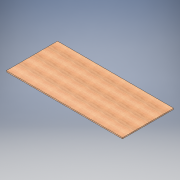
# Autodesk Inventor part: BedSlat
Saved by Autodesk Inventor 2017 (Build 210142000, 142)
## iProperties
Created: 2016-10-24
Part Number: BedSlat
Material: Generic
Document SubType Name: Modeling
Designer: andrew
Density: 1 g/cm^3
Appearance: Birch - Natural Polished
d1: 80.000 in
d2: 35.250 in
Author: andrew
Autodesk Inventor part; units mm, degrees
ref_plane "YZ Plane" through (0, 0, 0) normal (1, 0, 0) x (0, 1, 0)
ref_plane "XZ Plane" through (0, 0, 0) normal (0, 1, 0) x (-1, 0, 0)
ref_plane "XY Plane" through (0, 0, 0) normal (0, 0, 1) x (1, 0, 0)
sketch "Sketch1" plane through (0, 0, 0) normal (0, 1, 0) x (-1, 0, 0)
  line L0 (-1016, 447.675) -> (1016, 447.675)
  line L1 (1016, 447.675) -> (1016, -447.675)
  line L2 (1016, -447.675) -> (-1016, -447.675)
  line L3 (-1016, -447.675) -> (-1016, 447.675)
  line L4 (-1016, 447.675) -> (1016, -447.675) construction
  line L5 (1016, 447.675) -> (-1016, -447.675) construction
  point P0 (0, 0)
  dimension "d1" = 2032
  dimension "d2" = 895.35
  constraints: 12 end point, 2 midpoint, 2 parallel, 1 horizontal, 1 perpendicular
  measures "d1" distance of L0.start L0.end
  measures "d2" distance of L0.end L1.end
extrude "Extrusion1" add sketch "Sketch1" along normal blind 19.05
equation "\"d1\" = d0"
equation "\"d0\" = 2032"
body "Solid1"
